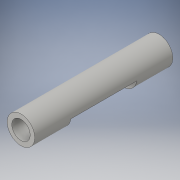
# Autodesk Inventor part: WireCounterPiece2
Saved by Autodesk Inventor 2016 (Build 200138000, 138)
## iProperties
Created: 2015-12-01
Part Number: WireCounterPiece2
Material: Generic
Document SubType Name: Modeling
Designer: Javier
Density: 1 g/cm^3
Appearance: Default
Author: Javier
Autodesk Inventor part; units mm, degrees
ref_plane "YZ Plane" through (0, 0, 0) normal (1, 0, 0) x (0, 1, 0)
ref_plane "XZ Plane" through (0, 0, 0) normal (0, 1, 0) x (-1, 0, 0)
ref_plane "XY Plane" through (0, 0, 0) normal (0, 0, 1) x (1, 0, 0)
sketch "Sketch1" plane through (0, 0, 0) normal (0, 0, 1) x (1, 0, 0)
  circle A0 centre (0, 0) radius 8.4667
  circle A1 centre (0, 0) radius 12.7
  dimension "d4" = 25.4
  constraints: 2 centre point, 2 coincident
  measures "d4" diameter of A1
extrude "Extrusion1" add sketch "Sketch1" along normal blind 127
sketch "Sketch2" plane through (0, 0, 0) normal (1, 0, 0) x (0, 1, 0)
  line L0 (-15.1143, 93.7374) -> (-1.5875, 93.7374)
  line L1 (-1.5875, 93.7374) -> (-1.5875, 33.1667)
  line L2 (-1.5875, 33.1667) -> (-15.1143, 33.1667)
  line L3 (-15.1143, 33.1667) -> (-15.1143, 93.7374)
  point P0 (0, 0)
  constraints: 8 end point, 2 parallel, 1 horizontal, 1 perpendicular
extrude "Extrusion2" cut sketch "Sketch2" along normal mid plane 76.2
body "Solid1"
